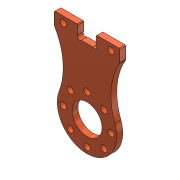
# Autodesk Inventor part: 16_008_COXA_FRAME_3_R1
Saved by Autodesk Inventor 2021.2 (Build 252289000, 289)
## iProperties
Created: 2018-04-27
Part Number: 16_008_COXA_FRAME_3_R1
Material: Aluminum 6061
Document SubType Name: Modeling
Designer: cmflab
Density: 2.7 g/cm^3
Appearance: Smooth - Light Orange
Mass: 1.00043 g
Surface Area: 14.2512 cm^2
Volume: 1.00043 cm^3
Author: cmflab
Autodesk Inventor part; units mm, degrees
ref_plane "YZ Plane" through (0, 0, 0) normal (1, 0, 0) x (0, 1, 0)
ref_plane "XZ Plane" through (0, 0, 0) normal (0, 1, 0) x (-1, 0, 0)
ref_plane "XY Plane" through (0, 0, 0) normal (0, 0, 1) x (1, 0, 0)
sketch "スケッチ1" plane through (0, 0, 0) normal (0, 1, 0) x (-1, 0, 0)
  line L0 (0, 0) -> (0, -24) construction
  circle A0 centre (0, -24) radius 5
  arc A1 (-9.3528, -20.4608) -> (9.3528, -20.4608) centre (0, -24) ccw
  line L1 (11, -2) -> (-11, -2) construction
  line L2 (-11, -2) -> (-11, 2)
  line L3 (11, 2) -> (11, -2)
  line L4 (11, 0) -> (-11, 0) construction
  circle A2 centre (8, 0) radius 1.05
  circle A3 centre (-8, 0) radius 1.05
  circle A4 centre (0, -24) radius 8 construction
  circle A5 centre (5.6569, -18.3431) radius 1.05
  circle A6 centre (0, -16) radius 1.05
  circle A7 centre (-5.6569, -18.3431) radius 1.05
  circle A8 centre (-8, -24) radius 1.05
  circle A9 centre (-5.6569, -29.6569) radius 1.05
  circle A10 centre (0, -32) radius 1.05
  circle A11 centre (5.6569, -29.6569) radius 1.05
  circle A12 centre (8, -24) radius 1.05
  line L5 (-3.05, 2) -> (-3.05, -0.9893)
  line L6 (-3.05, -2.05) -> (-1.9893, -2.05) construction
  arc A13 (1.9893, -2.05) -> (3.05, -0.9893) centre (2.5197, -1.5197) ccw
  line L7 (3.05, -2.05) -> (2.5197, -1.5197) construction
  line L8 (3.05, -0.9893) -> (3.05, 2)
  arc A14 (-3.05, -0.9893) -> (-1.9893, -2.05) centre (-2.5197, -1.5197) ccw
  line L9 (-3.05, -2.05) -> (-2.5197, -1.5197) construction
  line L10 (-3.05, -0.9893) -> (-3.05, -2.05) construction
  line L11 (-1.9893, -2.05) -> (1.9893, -2.05)
  line L12 (3.05, -0.9893) -> (3.05, -2.05) construction
  line L13 (1.9893, -2.05) -> (3.05, -2.05) construction
  line L14 (-11, 2) -> (-3.05, 2)
  line L15 (3.05, 2) -> (11, 2)
  arc A15 (10.863, -2.5052) -> (11, -2) centre (10, -2) ccw
  arc A16 (10.863, -2.5052) -> (9.3528, -20.4608) centre (28.9008, -13.0637) ccw
  line L16 (8, -6.3971) -> (8, -16.9723) construction
  arc A17 (-11, -2) -> (-10.863, -2.5052) centre (-10, -2) ccw
  arc A18 (-9.3528, -20.4608) -> (-10.863, -2.5052) centre (-28.9008, -13.0637) ccw
  dimension "d18" = 16
  dimension "d0" = 22
  dimension "d1" = 10
  dimension "d2" = 10
  dimension "d5" = 16
  dimension "d6" = 2.1
  dimension "d16" = 360
  dimension "d19" = 2.1
  dimension "d20" = 22
  dimension "d23" = 0.75
  dimension "d26" = 6.1
  dimension "d28" = 45
  dimension "d29" = 0.75
  dimension "d30" = 45
  dimension "d32" = 4
  dimension "d33" = 4.05
  dimension "d34" = 1
  dimension "d35" = 16
  constraints: 34 end point, 18 centre point, 16 point on circle, 7 parallel, 5 symmetric about line, 4 tangent, 3 coincident, 3 midpoint, 3 point on line, 2 horizontal, 2 vertical, 1 collinear, 1 equal radius, 1 perpendicular, 24 other
  measures "d0" distance of L3.start L2.end
  measures "d1" diameter of A0
  measures "d2" radius of A1
  measures "d5" distance of A2.centre A3.centre
  measures "d6" diameter of A2
  measures "d19" diameter of A6
  measures "d20" distance from line of L0.end L1
  measures "d23" radius of A13
  measures "d26" distance between parallel lines of L5 L8
  measures "d28" angle of L5 L9
  measures "d29" radius of A14
  measures "d30" angle of L12 L7
  measures "d32" diameter of L15 L4
  measures "d33" distance between parallel lines of L14 L11
  measures "d34" radius of A15
  measures "d35" diameter of L16 L0
extrude "押し出し1" add sketch "スケッチ1" along normal blind 2
chamfer "面取り1" distance 0.25 angle 45 4 edges at (11, 1, 2) (-11, 1, 2) (-3.05, 1, 2) (3.05, 1, 2)
